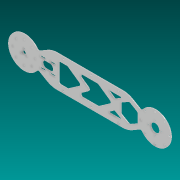
# Autodesk Inventor part: arm1v2
Saved by Autodesk Inventor 2020.3 (Build 243373000, 373)
## iProperties
Created: 2020-05-23
Part Number: arm1v2
Material: Aluminum 6061
Document SubType Name: Sheet Metal
Designer: Svend
Mass: 232.394 g
Surface Area: 513.63 cm^2
Volume: 86.0718 cm^3
Density: 2.7 g/cm^3
Sheet Metal Rule: Default_mm
Appearance: Aluminum - Polished
Author: Svend
Autodesk Inventor part; units mm, degrees
ref_plane "YZ Plane" through (0, 0, 0) normal (1, 0, 0) x (0, 1, 0)
ref_plane "XZ Plane" through (0, 0, 0) normal (0, 1, 0) x (-1, 0, 0)
ref_plane "XY Plane" through (0, 0, 0) normal (0, 0, 1) x (1, 0, 0)
sketch "Sketch1" plane through (0, 0, 0) normal (0, 0, 1) x (1, 0, 0)
  circle A0 centre (346.0004, 0) radius 1.55
  circle A1 centre (330, 0) radius 11
  arc A2 (51.9261, 10.7279) -> (51.9261, 14.7279) centre (51.9261, 12.7279) ccw
  line L0 (51.9261, 10.7279) -> (41.9261, 10.7279)
  arc A3 (41.9261, 14.7279) -> (41.9261, 10.7279) centre (41.9261, 12.7279) ccw
  line L1 (41.9261, 14.7279) -> (51.9261, 14.7279)
  arc A4 (77.3819, 10.7279) -> (77.3819, 14.7279) centre (77.3819, 12.7279) ccw
  line L2 (77.3819, 10.7279) -> (67.3819, 10.7279)
  arc A5 (67.3819, 14.7279) -> (67.3819, 10.7279) centre (67.3819, 12.7279) ccw
  line L3 (67.3819, 14.7279) -> (77.3819, 14.7279)
  arc A6 (51.9261, -14.7279) -> (51.9261, -10.7279) centre (51.9261, -12.7279) ccw
  line L4 (51.9261, -14.7279) -> (41.9261, -14.7279)
  arc A7 (41.9261, -10.7279) -> (41.9261, -14.7279) centre (41.9261, -12.7279) ccw
  line L5 (41.9261, -10.7279) -> (51.9261, -10.7279)
  arc A8 (67.3819, -10.7279) -> (67.3819, -14.7279) centre (67.3819, -12.7279) ccw
  line L6 (67.3819, -10.7279) -> (77.3819, -10.7279)
  arc A9 (77.3819, -14.7279) -> (77.3819, -10.7279) centre (77.3819, -12.7279) ccw
  line L7 (77.3819, -14.7279) -> (67.3819, -14.7279)
  circle A10 centre (59.654, 0) radius 8.5
  circle A11 centre (28, 0) radius 1.6
  line L8 (0, -40) -> (330, -40)
  arc A12 (330, -40) -> (330, 40) centre (330, 0) ccw
  line L9 (330, 40) -> (0, 40)
  arc A13 (0, 40) -> (0, -40) centre (0, 0) ccw
  line L10 (-4.8, -1) -> (-4.8, 1)
  line L11 (-4.8, 1) -> (-3.873, 1)
  arc A14 (-3.873, -1) -> (-3.873, 1) centre (0, 0) ccw
  line L12 (-3.873, -1) -> (-4.8, -1)
  circle A15 centre (0, 8) radius 2
  circle A16 centre (-6.9282, -4) radius 2
  circle A17 centre (6.9282, -4) radius 2
  circle A18 centre (19.799, 19.799) radius 1.6
  circle A19 centre (0, 28) radius 1.6
  circle A20 centre (-19.799, 19.799) radius 1.6
  circle A21 centre (-28, 0) radius 1.6
  circle A22 centre (-19.799, -19.799) radius 1.6
  circle A23 centre (0, -28) radius 1.6
  circle A24 centre (19.799, -19.799) radius 1.6
  circle A25 centre (330, 16.0004) radius 1.55
  circle A26 centre (313.9996, 0) radius 1.55
  circle A27 centre (330, -16.0004) radius 1.55
  line L13 (54.654, 0) -> (64.654, 0) construction
  line L14 (54.654, -8.5) -> (64.654, -8.5)
  line L15 (64.654, 8.5) -> (54.654, 8.5)
  arc A28 (54.654, 8.5) -> (54.654, -8.5) centre (54.654, 0) ccw
  arc A29 (64.654, -8.5) -> (64.654, 8.5) centre (64.654, 0) ccw
  point P0 (-4.8, 0)
  point P1 (4, 0)
  point P2 (370, 0)
  dimension "d0" = 4
  dimension "d1" = 8.8
  dimension "d2" = 2
  dimension "d6" = 4
  dimension "d7" = 8
  dimension "d14" = 360
  dimension "d16" = 28
  dimension "d17" = 3.2
  dimension "d20" = 360
  dimension "d22" = 17
  dimension "d23" = 59.654
  dimension "d24" = 2
  dimension "d25" = 10
  dimension "d26" = 12.7279
  dimension "d27" = 17.7279
  dimension "d28" = 12.7279
  dimension "d29" = 17.7279
  dimension "d30" = 17.7279
  dimension "d31" = 17.7279
  dimension "d32" = 22
  dimension "d33" = 39.9999
  dimension "d35" = 3.1
  dimension "d36" = 16.0004
  dimension "d39" = 360
  dimension "d72" = 270.346
  dimension "d87" = 5
  measures "d0" radius of A14
  measures "d1" distance from line of point (4, 0) L10
  measures "d2" distance between parallel lines of L12 L11
  measures "d6" diameter of A15
  measures "d7" distance of A14.centre A15.centre
  measures "d16" distance of A14.centre A11.centre
  measures "d17" diameter of A11
  measures "d22" diameter of A10
  measures "d23" distance of A14.centre A10.centre
  measures "d24" radius of A3
  measures "d25" distance of L0.start L0.end
  measures "d26" vertical distance of A10.centre A2.centre
  measures "d27" horizontal distance of A10.centre A3.centre
  measures "d28" vertical distance of A8.centre A10.centre
  measures "d29" horizontal distance of A9.centre A10.centre
  measures "d30" horizontal distance of A7.centre A10.centre
  measures "d31" horizontal distance of A4.centre A10.centre
  measures "d32" diameter of A1
  measures "d33" radius of A13
  measures "d35" diameter of A0
  measures "d36" distance of A1.centre A0.centre
  measures "d72" distance of A1.centre A10.centre
  measures "d87" distance of A10.centre L13.end
extrude "Plate1" add sketch "Sketch1" along normal mid plane 2
sketch "Sketch2" plane through (0, 0, -1) normal (0, 0, -1) x (-1, 0, 0)
  circle A0 centre (-330, 0) radius 11 projected
  line L0 (-77.3819, -10.7279) -> (-67.3819, -10.7279) projected
  arc A1 (-67.3819, -14.7279) -> (-67.3819, -10.7279) centre (-67.3819, -12.7279) ccw projected
  line L1 (-67.3819, -14.7279) -> (-77.3819, -14.7279) projected
  arc A2 (-77.3819, -10.7279) -> (-77.3819, -14.7279) centre (-77.3819, -12.7279) ccw projected
  line L2 (-41.9261, -14.7279) -> (-51.9261, -14.7279) projected
  arc A3 (-51.9261, -10.7279) -> (-51.9261, -14.7279) centre (-51.9261, -12.7279) ccw projected
  line L3 (-51.9261, -10.7279) -> (-41.9261, -10.7279) projected
  arc A4 (-41.9261, -14.7279) -> (-41.9261, -10.7279) centre (-41.9261, -12.7279) ccw projected
  line L4 (-67.3819, 10.7279) -> (-77.3819, 10.7279) projected
  arc A5 (-77.3819, 14.7279) -> (-77.3819, 10.7279) centre (-77.3819, 12.7279) ccw projected
  line L5 (-77.3819, 14.7279) -> (-67.3819, 14.7279) projected
  arc A6 (-67.3819, 10.7279) -> (-67.3819, 14.7279) centre (-67.3819, 12.7279) ccw projected
  line L6 (-41.9261, 10.7279) -> (-51.9261, 10.7279) projected
  arc A7 (-51.9261, 14.7279) -> (-51.9261, 10.7279) centre (-51.9261, 12.7279) ccw projected
  line L7 (-51.9261, 14.7279) -> (-41.9261, 14.7279) projected
  arc A8 (-41.9261, 10.7279) -> (-41.9261, 14.7279) centre (-41.9261, 12.7279) ccw projected
  line L8 (3.873, 1) -> (4.8, 1) projected
  line L9 (4.8, 1) -> (4.8, -1) projected
  line L10 (4.8, -1) -> (3.873, -1) projected
  arc A9 (3.873, 1) -> (3.873, -1) centre (0, 0) ccw projected
  circle A10 centre (-6.9282, -4) radius 2 projected
  circle A11 centre (6.9282, -4) radius 2 projected
  circle A12 centre (0, 8) radius 2 projected
  circle A13 centre (-19.799, -19.799) radius 1.6 projected
  circle A14 centre (0, -28) radius 1.6 projected
  circle A15 centre (19.799, -19.799) radius 1.6 projected
  circle A16 centre (28, 0) radius 1.6 projected
  circle A17 centre (19.799, 19.799) radius 1.6 projected
  circle A18 centre (0, 28) radius 1.6 projected
  circle A19 centre (-19.799, 19.799) radius 1.6 projected
  circle A20 centre (-28, 0) radius 1.6 projected
  circle A21 centre (-330, -16.0004) radius 1.55 projected
  circle A22 centre (-313.9996, 0) radius 1.55 projected
  circle A23 centre (-330, 16.0004) radius 1.55 projected
  circle A24 centre (-346.0004, 0) radius 1.55 projected
  line L11 (0, -40) -> (-330, -40) projected
  arc A25 (0, -40) -> (0, 40) centre (0, 0) ccw projected
  line L12 (-330, 40) -> (0, 40) projected
  arc A26 (-330, 40) -> (-330, -40) centre (-330, 0) ccw projected
  line L13 (-330, 40) -> (0, 40) projected
  arc A27 (-330, 40) -> (-330, -40) centre (-330, 0) ccw projected
  line L14 (-330, 0) -> (0, 0)
  line L15 (0, -40) -> (-330, -40) projected
  line L16 (-209.9233, -25) -> (-249.9233, -25)
  line L17 (-249.9233, -25) -> (-228, -12.3426)
  line L18 (-228, -12.3426) -> (-209.9233, -25)
  line L19 (-260.718, -40) -> (-295.359, -20)
  line L20 (-222, 0) -> (-186.2963, -25)
  line L21 (-186.2963, -25) -> (-131.2963, -25)
  line L22 (-131.2963, -25) -> (-167, 0)
  line L23 (-109.2963, -25) -> (-145, 0)
  line L24 (-87, -25) -> (-109.2963, -25)
  line L25 (-87, -25) -> (-87, 0)
  line L26 (-209.9233, 25) -> (-249.9233, 25)
  line L27 (-249.9233, 25) -> (-228, 12.3426)
  line L28 (-228, 12.3426) -> (-209.9233, 25)
  line L29 (-222, 0) -> (-186.2963, 25)
  line L30 (-186.2963, 25) -> (-131.2963, 25)
  line L31 (-131.2963, 25) -> (-167, 0)
  line L32 (-109.2963, 25) -> (-145, 0)
  line L33 (-87, 25) -> (-109.2963, 25)
  line L34 (-87, 25) -> (-87, 0)
  line L35 (-295.359, 20) -> (-260.718, 40)
  line L36 (-260.718, 40) -> (-330, 40)
  arc A28 (-295.359, 20) -> (-330, 40) centre (-330, 0) ccw
  arc A29 (-330, -40) -> (-295.359, -20) centre (-330, 0) ccw
  line L37 (-286.6506, -12.5) -> (-286.6506, 12.5)
  line L38 (-286.6506, 12.5) -> (-265, 25)
  line L39 (-265, 25) -> (-243.3494, 12.5)
  line L40 (-243.3494, 12.5) -> (-243.3494, -12.5)
  line L41 (-243.3494, -12.5) -> (-265, -25)
  line L42 (-265, -25) -> (-286.6506, -12.5)
  line L43 (-165, 40) -> (-165, -40)
  line L44 (0, 40) -> (-330, 40)
  line L45 (-69.282, -40) -> (-34.641, -20)
  arc A30 (-34.641, -20) -> (0, -40) centre (0, 0) ccw
  line L46 (-330, -40) -> (0, -40) projected
  line L47 (0, -40) -> (-69.282, -40)
  line L48 (-69.282, 40) -> (-34.641, 20)
  arc A31 (0, 40) -> (-34.641, 20) centre (0, 0) ccw
  line L49 (0, 40) -> (-69.282, 40)
  point P0 (-323.7858, 40)
  point P1 (-323.7858, -40)
  point P2 (-265, 0)
  point P3 (-228, 0)
  point P4 (-265, 0)
  dimension "d47" = 40
  dimension "d49" = 102
  dimension "d52" = 35
  dimension "d54" = 55
  dimension "d55" = 25
  dimension "d59" = 108
  dimension "d60" = 185
  dimension "d64" = 58
  dimension "d67" = 65
  constraints: 69 end point, 15 symmetric about line, 9 parallel, 9 point on line, 8 point on circle, 4 centre point, 4 collinear, 4 horizontal alignment, 4 line through centre, 3 coincident, 3 horizontal, 3 midpoint, 3 perpendicular, 3 tangent, 1 vertical alignment, 15 other
  measures "d47" distance of L16.start L16.end
  measures "d49" distance of A0.centre point (-228, 0)
  measures "d52" angle of L22 L21
  measures "d54" distance of L20.end L21.end
  measures "d55" distance between parallel lines of L14 L21
  measures "d59" distance of A0.centre L20.start
  measures "d60" distance of A0.centre L23.end
  measures "d64" distance from line of L25 L23.end
  measures "d67" distance of A0.centre point (-265, 0)
extrude "Cut1" cut sketch "Sketch2" against normal blind 2 contours L11 L45 A30 | A31 L48 L12 | L11 A29 L19 | L43 L22 L21 | L21 L20 L14 L22 L43 | L35 A28 L12 | L43 L31 L14 L29 L30 | L30 L31 L43 | L32 L33 L34 L14 | L14 L25 L24 L23 | L37 L38 L39 L40 L14 | L14 L40 L41 L42 L37 | L16 L17 L18 | L28 L27 L26
fillet "Fillet1" radius 2 6 edges at (249.9233, -25, 0) (209.9233, -25, 0) (228, -12.3426, 0) (249.9233, 25, 0) (228, 12.3426, 0) (209.9233, 25, 0)
fillet "Fillet2" radius 5 6 edges at (286.6506, -12.5, 0) (265, -25, 0) (243.3494, -12.5, 0) (243.3494, 12.5, 0) (265, 25, 0) (286.6506, 12.5, 0)
fillet "Fillet3" radius 5 11 edges at (222, 0, 0) (186.2963, -25, 0) (131.2963, -25, 0) (131.2963, 25, 0) (167, 0, 0) (186.2963, 25, 0) (145, 0, 0) (109.2963, -25, 0) (87, -25, 0) (87, 25, 0) (109.2963, 25, 0)
fillet "Fillet4" radius 50 4 edges at (260.718, -40, 0) (260.718, 40, 0) (69.282, 40, 0) (69.282, -40, 0)
fillet "Fillet5" radius 5 4 edges at (295.359, -20, 0) (295.359, 20, 0) (34.641, -20, 0) (34.641, 20, 0)
sketch "Sketch3" plane through (0, 0, -1) normal (0, 0, -1) x (-1, 0, 0)
  arc A0 (-82.6794, -40) -> (-57.6794, -33.3012) centre (-82.6794, 10) ccw projected
  line L0 (-57.6794, -33.3012) -> (-38.7298, -22.3607) projected
  arc A1 (-32.2043, -23.7251) -> (-38.7298, -22.3607) centre (-36.2298, -26.6908) ccw projected
  arc A2 (-32.2043, -23.7251) -> (-32.2043, 23.7251) centre (0, 0) ccw projected
  arc A3 (-38.7298, 22.3607) -> (-32.2043, 23.7251) centre (-36.2298, 26.6908) ccw projected
  line L1 (-38.7298, 22.3607) -> (-57.6794, 33.3012) projected
  arc A4 (-57.6794, 33.3012) -> (-82.6794, 40) centre (-82.6794, -10) ccw projected
  line L2 (-247.3206, 40) -> (-82.6794, 40) projected
  arc A5 (-247.3206, 40) -> (-272.3206, 33.3012) centre (-247.3206, -10) ccw projected
  line L3 (-272.3206, 33.3012) -> (-291.2702, 22.3607) projected
  arc A6 (-297.7957, 23.7251) -> (-291.2702, 22.3607) centre (-293.7702, 26.6908) ccw projected
  arc A7 (-297.7957, 23.7251) -> (-297.7957, -23.7251) centre (-330, 0) ccw projected
  arc A8 (-291.2702, -22.3607) -> (-297.7957, -23.7251) centre (-293.7702, -26.6908) ccw projected
  line L4 (-291.2702, -22.3607) -> (-272.3206, -33.3012) projected
  arc A9 (-272.3206, -33.3012) -> (-247.3206, -40) centre (-247.3206, 10) ccw projected
  line L5 (-82.6794, -40) -> (-247.3206, -40) projected
  arc A10 (-161.1506, 4.0958) -> (-161.1506, -4.0958) centre (-158.2828, 0) ccw projected
  line L6 (-161.1506, -4.0958) -> (-144.2864, -15.9042) projected
  arc A11 (-147.1543, -25) -> (-144.2864, -15.9042) centre (-147.1543, -20) ccw projected
  line L7 (-147.1543, -25) -> (-184.7198, -25) projected
  arc A12 (-187.5877, -24.0958) -> (-184.7198, -25) centre (-184.7198, -20) ccw projected
  line L8 (-187.5877, -24.0958) -> (-216.1506, -4.0958) projected
  arc A13 (-216.1506, 4.0958) -> (-216.1506, -4.0958) centre (-213.2828, 0) ccw projected
  line L9 (-216.1506, 4.0958) -> (-187.5877, 24.0958) projected
  arc A14 (-184.7198, 25) -> (-187.5877, 24.0958) centre (-184.7198, 20) ccw projected
  line L10 (-184.7198, 25) -> (-147.1543, 25) projected
  arc A15 (-144.2864, 15.9042) -> (-147.1543, 25) centre (-147.1543, 20) ccw projected
  line L11 (-144.2864, 15.9042) -> (-161.1506, 4.0958) projected
  line L12 (-215.1194, 21.3617) -> (-226.9563, 13.0734) projected
  arc A16 (-229.1034, 12.9796) -> (-226.9563, 13.0734) centre (-228.1034, 14.7117) ccw projected
  line L13 (-229.1034, 12.9796) -> (-243.4592, 21.2679) projected
  arc A17 (-242.4592, 25) -> (-243.4592, 21.2679) centre (-242.4592, 23) ccw projected
  line L14 (-242.4592, 25) -> (-216.2665, 25) projected
  arc A18 (-215.1194, 21.3617) -> (-216.2665, 25) centre (-216.2665, 23) ccw projected
  line L15 (-226.9563, -13.0734) -> (-215.1194, -21.3617) projected
  arc A19 (-216.2665, -25) -> (-215.1194, -21.3617) centre (-216.2665, -23) ccw projected
  line L16 (-216.2665, -25) -> (-242.4592, -25) projected
  arc A20 (-243.4592, -21.2679) -> (-242.4592, -25) centre (-242.4592, -23) ccw projected
  line L17 (-243.4592, -21.2679) -> (-229.1034, -12.9796) projected
  arc A21 (-226.9563, -13.0734) -> (-229.1034, -12.9796) centre (-228.1034, -14.7117) ccw projected
  line L18 (-267.5, -23.5566) -> (-284.1506, -13.9434) projected
  arc A22 (-286.6506, -9.6132) -> (-284.1506, -13.9434) centre (-281.6506, -9.6132) ccw projected
  line L19 (-286.6506, -9.6132) -> (-286.6506, 9.6132) projected
  arc A23 (-284.1506, 13.9434) -> (-286.6506, 9.6132) centre (-281.6506, 9.6132) ccw projected
  line L20 (-284.1506, 13.9434) -> (-267.5, 23.5566) projected
  arc A24 (-262.5, 23.5566) -> (-267.5, 23.5566) centre (-265, 19.2265) ccw projected
  line L21 (-262.5, 23.5566) -> (-245.8494, 13.9434) projected
  arc A25 (-243.3494, 9.6132) -> (-245.8494, 13.9434) centre (-248.3494, 9.6132) ccw projected
  line L22 (-243.3494, 9.6132) -> (-243.3494, -9.6132) projected
  arc A26 (-245.8494, -13.9434) -> (-243.3494, -9.6132) centre (-248.3494, -9.6132) ccw projected
  line L23 (-245.8494, -13.9434) -> (-262.5, -23.5566) projected
  arc A27 (-267.5, -23.5566) -> (-262.5, -23.5566) centre (-265, -19.2265) ccw projected
  line L24 (-92, -25) -> (-107.7198, -25) projected
  arc A28 (-110.5877, -24.0958) -> (-107.7198, -25) centre (-107.7198, -20) ccw projected
  line L25 (-110.5877, -24.0958) -> (-139.1506, -4.0958) projected
  arc A29 (-139.1506, 4.0958) -> (-139.1506, -4.0958) centre (-136.2828, 0) ccw projected
  line L26 (-139.1506, 4.0958) -> (-110.5877, 24.0958) projected
  arc A30 (-107.7198, 25) -> (-110.5877, 24.0958) centre (-107.7198, 20) ccw projected
  line L27 (-107.7198, 25) -> (-92, 25) projected
  arc A31 (-87, 20) -> (-92, 25) centre (-92, 20) ccw projected
  line L28 (-87, 20) -> (-87, -20) projected
  arc A32 (-92, -25) -> (-87, -20) centre (-92, -20) ccw projected
  circle A33 centre (-330, 0) radius 11 projected
  line L29 (-77.3819, -10.7279) -> (-67.3819, -10.7279) projected
  arc A34 (-67.3819, -14.7279) -> (-67.3819, -10.7279) centre (-67.3819, -12.7279) ccw projected
  line L30 (-67.3819, -14.7279) -> (-77.3819, -14.7279) projected
  arc A35 (-77.3819, -10.7279) -> (-77.3819, -14.7279) centre (-77.3819, -12.7279) ccw projected
  line L31 (-41.9261, -14.7279) -> (-51.9261, -14.7279) projected
  arc A36 (-51.9261, -10.7279) -> (-51.9261, -14.7279) centre (-51.9261, -12.7279) ccw projected
  line L32 (-51.9261, -10.7279) -> (-41.9261, -10.7279) projected
  arc A37 (-41.9261, -14.7279) -> (-41.9261, -10.7279) centre (-41.9261, -12.7279) ccw projected
  line L33 (-67.3819, 10.7279) -> (-77.3819, 10.7279) projected
  arc A38 (-77.3819, 14.7279) -> (-77.3819, 10.7279) centre (-77.3819, 12.7279) ccw projected
  line L34 (-77.3819, 14.7279) -> (-67.3819, 14.7279) projected
  arc A39 (-67.3819, 10.7279) -> (-67.3819, 14.7279) centre (-67.3819, 12.7279) ccw projected
  line L35 (-41.9261, 10.7279) -> (-51.9261, 10.7279) projected
  arc A40 (-51.9261, 14.7279) -> (-51.9261, 10.7279) centre (-51.9261, 12.7279) ccw projected
  line L36 (-51.9261, 14.7279) -> (-41.9261, 14.7279) projected
  arc A41 (-41.9261, 10.7279) -> (-41.9261, 14.7279) centre (-41.9261, 12.7279) ccw projected
  line L37 (3.873, 1) -> (4.8, 1) projected
  line L38 (4.8, 1) -> (4.8, -1) projected
  line L39 (4.8, -1) -> (3.873, -1) projected
  arc A42 (3.873, 1) -> (3.873, -1) centre (0, 0) ccw projected
  circle A43 centre (-6.9282, -4) radius 2 projected
  circle A44 centre (6.9282, -4) radius 2 projected
  circle A45 centre (0, 8) radius 2 projected
  circle A46 centre (-19.799, -19.799) radius 1.6 projected
  circle A47 centre (0, -28) radius 1.6 projected
  circle A48 centre (19.799, -19.799) radius 1.6 projected
  circle A49 centre (28, 0) radius 1.6 projected
  circle A50 centre (19.799, 19.799) radius 1.6 projected
  circle A51 centre (0, 28) radius 1.6 projected
  circle A52 centre (-19.799, 19.799) radius 1.6 projected
  circle A53 centre (-28, 0) radius 1.6 projected
  circle A54 centre (-330, -16.0004) radius 1.55 projected
  circle A55 centre (-313.9996, 0) radius 1.55 projected
  circle A56 centre (-330, 16.0004) radius 1.55 projected
  circle A57 centre (-346.0004, 0) radius 1.55 projected
  circle A58 centre (-365.5, 0) radius 1.5
  circle A59 centre (-355.1023, -25.1023) radius 1.5
  circle A60 centre (-330, -35.5) radius 1.5
  circle A61 centre (-304.8977, -25.1023) radius 1.5
  circle A62 centre (-294.5, 0) radius 1.5
  circle A63 centre (-304.8977, 25.1023) radius 1.5
  circle A64 centre (-330, 35.5) radius 1.5
  circle A65 centre (-355.1023, 25.1023) radius 1.5
  point P0 (0, 0)
  dimension "d73" = 3
  dimension "d74" = 35.5
  dimension "d77" = 360
  constraints: 8 centre point, 1 horizontal alignment, 17 other
  measures "d73" diameter of A58
  measures "d74" distance of A33.centre A58.centre
chamfer "Chamfer2" distance 1.5 angle 45 4 edges at (344.4504, 0, -1) (328.45, 16.0004, -1) (312.4496, 0, -1) (328.45, -16.0004, -1)
hole "Hole1" at (330, -35.5, -1) at (355.1023, -25.1023, -1) at (365.5, 0, -1) at (355.1023, 25.1023, -1) at (330, 35.5, -1) at (304.8977, 25.1023, -1) at (294.5, 0, -1) at (304.8977, -25.1023, -1) direction (0, 0, 1) diameter 4 end through all clearance for "Countersunk Flat Head Screw ISO 2009/7046" size "M4" standard "ISO"
sketch "Sketch4" plane through (0, 0, 1) normal (0, 0, 1) x (1, 0, 0)
  circle A0 centre (294.5, 0) radius 2 projected
  circle A1 centre (330, 35.5) radius 2 projected
  circle A2 centre (365.5, 0) radius 2 projected
  circle A3 centre (330, -35.5) radius 2 projected
  circle A4 centre (355.1023, -25.1023) radius 2 projected
  circle A5 centre (355.1023, 25.1023) radius 2 projected
  circle A6 centre (304.8977, 25.1023) radius 2 projected
  circle A7 centre (304.8977, -25.1023) radius 2 projected
  arc A8 (57.6794, -33.3012) -> (82.6794, -40) centre (82.6794, 10) ccw projected
  line L0 (247.3206, -40) -> (82.6794, -40) projected
  arc A9 (247.3206, -40) -> (272.3206, -33.3012) centre (247.3206, 10) ccw projected
  line L1 (272.3206, -33.3012) -> (291.2702, -22.3607) projected
  arc A10 (297.7957, -23.7251) -> (291.2702, -22.3607) centre (293.7702, -26.6908) ccw projected
  arc A11 (297.7957, -23.7251) -> (297.7957, 23.7251) centre (330, 0) ccw projected
  arc A12 (291.2702, 22.3607) -> (297.7957, 23.7251) centre (293.7702, 26.6908) ccw projected
  line L2 (291.2702, 22.3607) -> (272.3206, 33.3012) projected
  arc A13 (272.3206, 33.3012) -> (247.3206, 40) centre (247.3206, -10) ccw projected
  line L3 (82.6794, 40) -> (247.3206, 40) projected
  arc A14 (82.6794, 40) -> (57.6794, 33.3012) centre (82.6794, -10) ccw projected
  line L4 (57.6794, 33.3012) -> (38.7298, 22.3607) projected
  arc A15 (32.2043, 23.7251) -> (38.7298, 22.3607) centre (36.2298, 26.6908) ccw projected
  arc A16 (32.2043, 23.7251) -> (32.2043, -23.7251) centre (0, 0) ccw projected
  arc A17 (38.7298, -22.3607) -> (32.2043, -23.7251) centre (36.2298, -26.6908) ccw projected
  line L5 (38.7298, -22.3607) -> (57.6794, -33.3012) projected
  line L6 (226.9563, 13.0734) -> (215.1194, 21.3617) projected
  arc A18 (216.2665, 25) -> (215.1194, 21.3617) centre (216.2665, 23) ccw projected
  line L7 (216.2665, 25) -> (242.4592, 25) projected
  arc A19 (243.4592, 21.2679) -> (242.4592, 25) centre (242.4592, 23) ccw projected
  line L8 (243.4592, 21.2679) -> (229.1034, 12.9796) projected
  arc A20 (226.9563, 13.0734) -> (229.1034, 12.9796) centre (228.1034, 14.7117) ccw projected
  arc A21 (161.1506, -4.0958) -> (161.1506, 4.0958) centre (158.2828, 0) ccw projected
  line L9 (161.1506, 4.0958) -> (144.2864, 15.9042) projected
  arc A22 (147.1543, 25) -> (144.2864, 15.9042) centre (147.1543, 20) ccw projected
  line L10 (147.1543, 25) -> (184.7198, 25) projected
  arc A23 (187.5877, 24.0958) -> (184.7198, 25) centre (184.7198, 20) ccw projected
  line L11 (187.5877, 24.0958) -> (216.1506, 4.0958) projected
  arc A24 (216.1506, -4.0958) -> (216.1506, 4.0958) centre (213.2828, 0) ccw projected
  line L12 (216.1506, -4.0958) -> (187.5877, -24.0958) projected
  arc A25 (184.7198, -25) -> (187.5877, -24.0958) centre (184.7198, -20) ccw projected
  line L13 (184.7198, -25) -> (147.1543, -25) projected
  arc A26 (144.2864, -15.9042) -> (147.1543, -25) centre (147.1543, -20) ccw projected
  line L14 (144.2864, -15.9042) -> (161.1506, -4.0958) projected
  line L15 (215.1194, -21.3617) -> (226.9563, -13.0734) projected
  arc A27 (229.1034, -12.9796) -> (226.9563, -13.0734) centre (228.1034, -14.7117) ccw projected
  line L16 (229.1034, -12.9796) -> (243.4592, -21.2679) projected
  arc A28 (242.4592, -25) -> (243.4592, -21.2679) centre (242.4592, -23) ccw projected
  line L17 (242.4592, -25) -> (216.2665, -25) projected
  arc A29 (215.1194, -21.3617) -> (216.2665, -25) centre (216.2665, -23) ccw projected
  line L18 (284.1506, -13.9434) -> (267.5, -23.5566) projected
  arc A30 (262.5, -23.5566) -> (267.5, -23.5566) centre (265, -19.2265) ccw projected
  line L19 (262.5, -23.5566) -> (245.8494, -13.9434) projected
  arc A31 (243.3494, -9.6132) -> (245.8494, -13.9434) centre (248.3494, -9.6132) ccw projected
  line L20 (243.3494, -9.6132) -> (243.3494, 9.6132) projected
  arc A32 (245.8494, 13.9434) -> (243.3494, 9.6132) centre (248.3494, 9.6132) ccw projected
  line L21 (245.8494, 13.9434) -> (262.5, 23.5566) projected
  arc A33 (267.5, 23.5566) -> (262.5, 23.5566) centre (265, 19.2265) ccw projected
  line L22 (267.5, 23.5566) -> (284.1506, 13.9434) projected
  arc A34 (286.6506, 9.6132) -> (284.1506, 13.9434) centre (281.6506, 9.6132) ccw projected
  line L23 (286.6506, 9.6132) -> (286.6506, -9.6132) projected
  arc A35 (284.1506, -13.9434) -> (286.6506, -9.6132) centre (281.6506, -9.6132) ccw projected
  line L24 (107.7198, -25) -> (92, -25) projected
  arc A36 (87, -20) -> (92, -25) centre (92, -20) ccw projected
  line L25 (87, -20) -> (87, 20) projected
  arc A37 (92, 25) -> (87, 20) centre (92, 20) ccw projected
  line L26 (92, 25) -> (107.7198, 25) projected
  arc A38 (110.5877, 24.0958) -> (107.7198, 25) centre (107.7198, 20) ccw projected
  line L27 (110.5877, 24.0958) -> (139.1506, 4.0958) projected
  arc A39 (139.1506, -4.0958) -> (139.1506, 4.0958) centre (136.2828, 0) ccw projected
  line L28 (139.1506, -4.0958) -> (110.5877, -24.0958) projected
  arc A40 (107.7198, -25) -> (110.5877, -24.0958) centre (107.7198, -20) ccw projected
  arc A41 (54.654, 8.5) -> (54.654, -8.5) centre (54.654, 0) ccw projected
  line L29 (54.654, 8.5) -> (64.654, 8.5) projected
  arc A42 (64.654, -8.5) -> (64.654, 8.5) centre (64.654, 0) ccw projected
  line L30 (64.654, -8.5) -> (54.654, -8.5) projected
  circle A43 centre (330, 0) radius 11 projected
  line L31 (67.3819, -10.7279) -> (77.3819, -10.7279) projected
  arc A44 (77.3819, -14.7279) -> (77.3819, -10.7279) centre (77.3819, -12.7279) ccw projected
  line L32 (77.3819, -14.7279) -> (67.3819, -14.7279) projected
  arc A45 (67.3819, -10.7279) -> (67.3819, -14.7279) centre (67.3819, -12.7279) ccw projected
  line L33 (51.9261, -14.7279) -> (41.9261, -14.7279) projected
  arc A46 (41.9261, -10.7279) -> (41.9261, -14.7279) centre (41.9261, -12.7279) ccw projected
  line L34 (41.9261, -10.7279) -> (51.9261, -10.7279) projected
  arc A47 (51.9261, -14.7279) -> (51.9261, -10.7279) centre (51.9261, -12.7279) ccw projected
  line L35 (77.3819, 10.7279) -> (67.3819, 10.7279) projected
  arc A48 (67.3819, 14.7279) -> (67.3819, 10.7279) centre (67.3819, 12.7279) ccw projected
  line L36 (67.3819, 14.7279) -> (77.3819, 14.7279) projected
  arc A49 (77.3819, 10.7279) -> (77.3819, 14.7279) centre (77.3819, 12.7279) ccw projected
  line L37 (51.9261, 10.7279) -> (41.9261, 10.7279) projected
  arc A50 (41.9261, 14.7279) -> (41.9261, 10.7279) centre (41.9261, 12.7279) ccw projected
  line L38 (41.9261, 14.7279) -> (51.9261, 14.7279) projected
  arc A51 (51.9261, 10.7279) -> (51.9261, 14.7279) centre (51.9261, 12.7279) ccw projected
  line L39 (-4.8, 1) -> (-3.873, 1) projected
  arc A52 (-3.873, -1) -> (-3.873, 1) centre (0, 0) ccw projected
  line L40 (-3.873, -1) -> (-4.8, -1) projected
  line L41 (-4.8, -1) -> (-4.8, 1) projected
  circle A53 centre (6.9282, -4) radius 2 projected
  circle A54 centre (-6.9282, -4) radius 2 projected
  circle A55 centre (0, 8) radius 2 projected
  circle A56 centre (19.799, -19.799) radius 1.6 projected
  circle A57 centre (0, -28) radius 1.6 projected
  circle A58 centre (-19.799, -19.799) radius 1.6 projected
  circle A59 centre (-28, 0) radius 1.6 projected
  circle A60 centre (-19.799, 19.799) radius 1.6 projected
  circle A61 centre (0, 28) radius 1.6 projected
  circle A62 centre (19.799, 19.799) radius 1.6 projected
  circle A63 centre (28, 0) radius 1.6 projected
  circle A64 centre (330, -16.0004) radius 1.55 projected
  circle A65 centre (313.9996, 0) radius 1.55 projected
  circle A66 centre (330, 16.0004) radius 1.55 projected
  circle A67 centre (346.0004, 0) radius 1.55 projected
  point P0 (0, 0)
  point P1 (99, 35)
  point P2 (169, 35)
  point P3 (239, 35)
  point P4 (99, -35)
  point P5 (169, -35)
  point P6 (239, -35)
  dimension "d95" = 5
  dimension "d96" = 5
  dimension "d97" = 12
  dimension "d98" = 70
  dimension "d99" = 70
  constraints: 4 horizontal alignment, 3 vertical alignment
  measures "d95" distance from line of L3 point (99, 35)
  measures "d96" distance from line of L0 point (99, -35)
  measures "d97" distance from line of L25 point (99, -35)
  measures "d98" distance of point (169, -35) point (99, -35)
  measures "d99" distance of point (239, -35) point (169, -35)
hole "Hole2" at (99, 35, 1) at (169, 35, 1) at (239, 35, 1) at (99, -35, 1) at (169, -35, 1) at (239, -35, 1) direction (0, 0, -1) diameter 4.2 end through all clearance for "Countersunk Flat Head Screw ISO 2009/7046" size "M4" standard "ISO"
equation "\"d41\" = Thickness"
equation "\"BendRadius\" = Thickness"
equation "\"BendReliefWidth\" = Thickness"
equation "\"CornerReliefSize\" = 4 * Thickness"
equation "\"TransitionRadius\" = BendRadius"
equation "\"JacobiRadiusSize\" = BendRadius"
equation "\"GapSize\" = Thickness"
equation "\"Thickness\" = 2"
body "Solid1"
